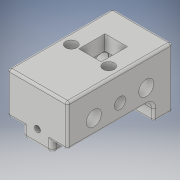
# Autodesk Inventor part: Y_Slider_Part
Saved by Autodesk Inventor 2019 (Build 230136000, 136)
## iProperties
Created: 2018-08-19
Part Number: Y_Slider_Part
Material: Generic
Document SubType Name: Modeling
Designer: Julia
Density: 1 g/cm^3
Appearance: Default
Author: Julia
Autodesk Inventor part; units mm, degrees
ref_plane "YZ Plane" through (0, 0, 0) normal (1, 0, 0) x (0, 1, 0)
ref_plane "XZ Plane" through (0, 0, 0) normal (0, 1, 0) x (-1, 0, 0)
ref_plane "XY Plane" through (0, 0, 0) normal (0, 0, 1) x (1, 0, 0)
sketch "Sketch1" plane through (0, 0, 0) normal (0, 1, 0) x (-1, 0, 0)
  line L0 (40, 70) -> (-40, 70)
  line L1 (-40, 70) -> (-40, -70)
  line L2 (-40, -70) -> (40, -70)
  line L3 (40, -70) -> (40, 70)
  point P0 (0, 0)
  point P1 (40, 0)
  point P2 (0, 70)
  dimension "d0" = 140
  dimension "d1" = 80
  constraints: 8 end point, 2 midpoint, 2 parallel, 1 horizontal, 1 horizontal alignment, 1 perpendicular, 1 vertical alignment
  measures "d0" distance of L2.end L0.start
  measures "d1" distance of L1.end L2.end
extrude "Extrusion1" add sketch "Sketch1" along normal blind 20
sketch "Sketch5" plane through (0, 20, 0) normal (0, 1, 0) x (1, 0, 0)
  line L0 (15, 35) -> (-15, 35)
  line L1 (-15, 35) -> (-15, 0)
  line L2 (-15, 0) -> (15, 0)
  line L3 (15, 0) -> (15, 35)
  point P0 (0, 0)
  point P1 (15, 17.5)
  point P2 (0, 35)
  dimension "d30" = 35
  dimension "d31" = 30
  constraints: 8 end point, 3 midpoint, 2 parallel, 1 horizontal, 1 perpendicular, 1 vertical alignment
  measures "d30" distance of L2.end L0.start
  measures "d31" distance of L1.end L2.end
extrude "Extrusion4" cut sketch "Sketch5" against normal blind 20
sketch "Sketch12" plane through (0, 0, 0) normal (0, -1, 0) x (1, 0, 0)
  line L0 (-40, 55) -> (-20, 55)
  line L1 (-20, 55) -> (-20, -55)
  line L2 (-20, -55) -> (-40, -55)
  line L3 (-40, -55) -> (-40, 55)
  line L4 (-40, -70) -> (-40, 70) projected
  line L5 (-15, 0) -> (15, 0) projected
  line L6 (0, 100.8809) -> (0, -116.5773) construction
  line L7 (40, 55) -> (20, 55)
  line L8 (20, 55) -> (20, -55)
  line L9 (20, -55) -> (40, -55)
  line L10 (40, -55) -> (40, 55)
  point P0 (0, 0)
  point P1 (-40, 0)
  point P2 (0, 0)
  dimension "d56" = 20
  dimension "d57" = 110
  constraints: 18 end point, 4 symmetric about line, 2 midpoint, 2 parallel, 2 vertical, 1 collinear, 1 horizontal, 1 horizontal alignment, 1 perpendicular
  measures "d56" distance of L0.start L0.end
  measures "d57" distance between parallel lines of L2 L0
extrude "Extrusion11" add sketch "Sketch12" along normal blind 35
sketch "Sketch13" plane through (-40, 0, 70) normal (-1, 0, 0) x (0, 0, 1)
  line L0 (-15, 0) -> (0, 0) projected
  line L1 (-15, 0) -> (-125, 0) projected
  point P0 (-70, 0)
  point P1 (-35, -15)
  point P2 (-105, -15)
  point P3 (-70, -15)
  point P4 (-70, 0)
  dimension "d60" = 15
  dimension "d61" = 35
  dimension "d62" = 35
  constraints: 2 horizontal alignment, 1 midpoint, 1 vertical alignment
  measures "d60" distance from line of point (-35, -15) L0
  measures "d61" horizontal distance of point (-70, 0) point (-35, -15)
  measures "d62" horizontal distance of point (-70, 0) point (-105, -15)
hole "Hole2" at (-40, -15, 35) at (-40, -15, -35) direction (1, 0, 0) diameter 20 end through all
hole "Hole3" at (-40, -15, 0) direction (1, 0, 0) diameter 15 end through all
sketch "Sketch14" plane through (0, 0, 0) normal (0, -1, 0) x (1, 0, 0)
  line L0 (40, -45) -> (-40, -45)
  line L1 (-40, -45) -> (-40, -70)
  line L2 (-40, -70) -> (40, -70)
  line L3 (40, -70) -> (40, -45)
  line L4 (40, -55) -> (40, -70) projected
  line L5 (40, -70) -> (-40, -70) projected
  line L6 (-40, -70) -> (-40, -55) projected
  line L7 (-15, 0) -> (15, 0) projected
  point P0 (0, 0)
  dimension "d77" = 45
  constraints: 8 end point, 3 collinear, 2 parallel, 1 horizontal, 1 perpendicular
  measures "d77" distance between parallel lines of L0 L7
extrude "Extrusion12" add sketch "Sketch14" along normal blind 60
fillet "Fillet10" radius 10 2 edges at (30, -35, -45) (-30, -35, -45)
sketch "Sketch15" plane through (-20, 0, -45) normal (0, 0, 1) x (1, 0, 0)
  line L0 (0, 0) -> (40, 0) projected
  line L1 (60, -60) -> (-20, -60) projected
  point P0 (20, 0)
  point P1 (20, -30)
  point P2 (20, -60)
  dimension "d82" = 30
  constraints: 1 midpoint, 1 vertical alignment
  measures "d82" distance from line of L0 point (20, -30)
hole "Hole4" at (0, -30, -45) direction (0, 0, -1) diameter 8 end through all both
sketch "Sketch16" plane through (0, 0, 0) normal (0, -1, 0) x (1, 0, 0)
  line L0 (20, 70) -> (-20, 70)
  line L1 (-20, 70) -> (-20, 45)
  line L2 (-20, 45) -> (20, 45)
  line L3 (20, 45) -> (20, 70)
  line L4 (-40, 70) -> (40, 70) projected
  line L5 (20, -45) -> (20, 55) projected
  line L6 (-20, 55) -> (-20, -45) projected
  line L7 (-15, 0) -> (15, 0) projected
  point P0 (0, 0)
  point P1 (20, 65)
  point P2 (-20, 65)
  dimension "d91" = 45
  constraints: 8 end point, 3 collinear, 2 parallel, 1 horizontal, 1 perpendicular
  measures "d91" distance between parallel lines of L7 L2
extrude "Extrusion13" add sketch "Sketch16" along normal blind 50
sketch "Sketch17" plane through (20, 0, 45) normal (0, 0, -1) x (-1, 0, 0)
  line L0 (40, -50) -> (0, -50) projected
  line L1 (0, 0) -> (40, 0) projected
  point P0 (20, 0)
  point P1 (20, -30)
  point P2 (20, -50)
  dimension "d94" = 30
  constraints: 1 midpoint, 1 vertical alignment
  measures "d94" distance from line of L1 point (20, -30)
hole "Hole5" at (0, -30, 45) direction (0, 0, 1) diameter 8 end through all both
fillet "Fillet12" radius 5 4 edges at (0, -50, 45) (20, -50, 57.5) (-20, -50, 57.5) (0, -50, 70)
fillet "Fillet13" radius 5 4 edges at (-18.5355, -48.5355, 46.4645) (-20, -40, 45) (18.5355, -48.5355, 46.4645) (20, -40, 45)
fillet "Fillet14" radius 5 4 edges at (18.5355, -48.5355, 68.5355) (20, -22.5, 70) (-18.5355, -48.5355, 68.5355) (-20, -22.5, 70)
sketch "Sketch18" plane through (0, 0, 0) normal (0, -1, 0) x (1, 0, 0)
  line L0 (40, 55) -> (15, 55)
  line L1 (15, 55) -> (15, 70)
  line L2 (15, 70) -> (40, 70)
  line L3 (40, 70) -> (40, 55)
  line L4 (15, 70) -> (40, 70) projected
  line L5 (40, 70) -> (40, 55) projected
  line L6 (20, 55) -> (40, 55) projected
  line L7 (-15, 55) -> (-40, 55)
  line L8 (-40, 55) -> (-40, 70)
  line L9 (-40, 70) -> (-15, 70)
  line L10 (-15, 70) -> (-15, 55)
  line L11 (-40, 55) -> (-20, 55) projected
  line L12 (-40, 55) -> (-40, 70) projected
  line L13 (-40, 70) -> (-15, 70) projected
  point P0 (0, 0)
  constraints: 16 end point, 6 collinear, 4 parallel, 2 horizontal, 2 perpendicular, 2 point on line
extrude "Extrusion14" add sketch "Sketch18" along normal blind 35
fillet "Fillet15" radius 3 13 edges at (-27.5, -35, 70) (27.5, -35, 70) (-40, -37.9289, -42.0711) (-40, -52.5, -45) (-40, -35, 17.5) (-20, -37.9289, -42.0711) (-20, -35, 5) (20, -37.9289, -42.0711) (20, -35, 5) (40, -37.9289, -42.0711) (40, -52.5, -45) (40, -35, 17.5) (0, -60, -45)
fillet "Fillet16" radius 3 2 edges at (-19, -35, 45) (19, -35, 45)
fillet "Fillet18" radius 3 15 edges at (39.1213, -59.1213, -45.8787) (40, -60, -59) (0, -60, -70) (-40, -20, -70) (-39.1213, -59.1213, -45.8787) (-40, -60, -59) (40, -20, -70) (40, 20, 0) (0, 20, -70) (0, 20, 70) (-39.1213, -34.1213, 69.1213) (-40, -6, 70) (-40, 20, 0) (39.1213, -34.1213, 69.1213) (40, -6, 70)
sketch "Sketch19" plane through (0, 20, 0) normal (0, 1, 0) x (1, 0, 0)
  point P0 (0, 0)
  point P1 (25, 0)
  point P2 (-25, 0)
  dimension "d111" = 25
  dimension "d112" = 25
  constraints: 2 horizontal alignment
  measures "d111" distance of point (0, 0) point (25, 0)
  measures "d112" distance of point (-25, 0) point (0, 0)
hole "Hole6" at (25, 20, 0) at (-25, 20, 0) direction (0, -1, 0) diameter 15 depth 15
body "Solid1"
